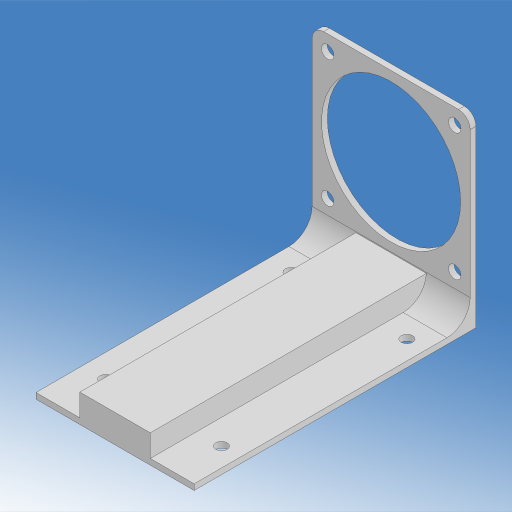
# Autodesk Inventor part: MotorStandoff
Saved by Autodesk Inventor 2024 (Build 280153000, 153)
## iProperties
Created: 2024-02-28
Part Number: MotorStandoff
Material: Generic
Document SubType Name: Modeling
Designer: seene
Density: 1 g/cm^3
Appearance: Default
Author: seene
Autodesk Inventor part; units mm, degrees
ref_plane "YZ Plane" through (0, 0, 0) normal (1, 0, 0) x (0, 1, 0)
ref_plane "XZ Plane" through (0, 0, 0) normal (0, 1, 0) x (-1, 0, 0)
ref_plane "XY Plane" through (0, 0, 0) normal (0, 0, 1) x (1, 0, 0)
sketch "Sketch1" plane through (0, 0, 0) normal (0, 1, 0) x (-1, 0, 0)
  line L0 (0, 0) -> (-86.614, 0)
  line L1 (-86.614, 0) -> (-86.614, -154.432)
  line L2 (-86.614, -154.432) -> (0, -154.432)
  line L3 (0, -154.432) -> (0, 0)
  circle A0 centre (-12.7, -25.4) radius 3.175
  circle A1 centre (-12.7, -127) radius 3.175
  circle A2 centre (-76.2, -25.4) radius 3.175
  circle A3 centre (-76.2, -127) radius 3.175
  line L4 (0, -154.432) -> (-86.614, -154.432)
  line L5 (-86.614, -154.432) -> (-86.614, -151.257)
  line L6 (-86.614, -151.257) -> (0, -151.257)
  line L7 (0, -151.257) -> (0, -154.432)
  point P0 (0, -151.257)
  dimension "d0" = 6.35
  dimension "d1" = 154.432
  dimension "d2" = 86.614
  dimension "d3" = 12.7
  dimension "d4" = 25.4
  dimension "d7" = 101.6
  dimension "d10" = 63.5
  dimension "d31" = 3.175
  constraints: 16 end point, 4 centre point, 4 parallel, 3 horizontal, 2 perpendicular, 1 point on line, 1 vertical, 6 other
  measures "d0" diameter of A0
  measures "d1" distance of L0.end L1.end
  measures "d2" distance of L0.start L0.end
  measures "d3" distance from line of A0.centre L3
  measures "d4" distance from line of L0 A0.centre
  measures "d7" distance of A0.centre A1.centre
  measures "d10" distance of A0.centre A2.centre
  measures "d31" distance between parallel lines of L2 L6
extrude "Extrusion1" add sketch "Sketch1" along normal blind 3.175 contours L3 L6 L1 L0
sketch "Sketch3" plane through (0, 3.175, 0) normal (0, 1, 0) x (1, 0, 0)
  line L0 (0, 0) -> (86.614, 0) projected
  line L1 (24.003, 0) -> (62.611, 0)
  line L2 (62.611, 0) -> (62.611, 151.257)
  line L3 (62.611, 151.257) -> (24.003, 151.257)
  line L4 (24.003, 151.257) -> (24.003, 0)
  line L5 (0, 151.257) -> (0, 0) projected
  line L6 (86.614, 0) -> (86.614, 151.257) projected
  line L7 (43.307, 0) -> (43.307, 154.432) construction
  line L8 (86.614, 154.432) -> (0, 154.432) construction
  line L9 (43.307, 0) -> (43.307, 151.257) construction
  line L10 (86.614, 151.257) -> (0, 151.257) projected
  dimension "d28" = 38.608
  constraints: 12 end point, 5 midpoint, 2 parallel, 2 point on line, 1 horizontal, 1 perpendicular
  measures "d28" distance between parallel lines of L2 L4
extrude "Extrusion3" add sketch "Sketch3" along normal blind 12.192 contours L4 L3 L2 L0
extrude "Extrusion4" add sketch "Sketch1" along normal blind 101.981 contours L3 L2 L1 L6
sketch "Sketch4" plane through (86.614, 0, -154.432) normal (0, 0, -1) x (-1, 0, 0)
  circle A0 centre (43.3338, 58.6472) radius 38.1
  circle A1 centre (8.5085, 93.4725) radius 3.4925
  line L0 (0, 0) -> (0, 101.981) projected
  line L1 (0, 101.981) -> (86.614, 101.981) projected
  circle A2 centre (78.1055, 93.4725) radius 3.4925
  circle A3 centre (8.5085, 23.8755) radius 3.4925
  circle A4 centre (78.1055, 23.8755) radius 3.4925
  point P0 (86.614, 0)
  dimension "d34" = 76.2
  dimension "d35" = 6.985
  dimension "d36" = 8.5085
  dimension "d38" = 8.5085
  dimension "d41" = 69.597
  dimension "d44" = 69.597
  dimension "d47" = 43.3338
  dimension "d48" = 43.3338
  constraints: 5 centre point, 1 horizontal, 1 vertical, 6 other
  measures "d34" diameter of A0
  measures "d35" diameter of A1
  measures "d36" distance from line of L0 A1.centre
  measures "d38" distance from line of L1 A1.centre
  measures "d41" distance of A1.centre A2.centre
  measures "d44" distance of A1.centre A3.centre
  measures "d47" distance from line of L1 A0.centre
  measures "d48" distance from line of L0 A0.centre
extrude "Extrusion5" cut sketch "Sketch4" against normal through all
fillet "Fillet1" radius 12.7 2 edges at (74.6125, 3.175, -151.257) (12.0015, 3.175, -151.257)
fillet "Fillet2" radius 6.35 2 edges at (86.614, 101.981, -152.8445) (0, 101.981, -152.8445)
equation "\"d28\" = 0.25 * d1"
body "Solid1"
